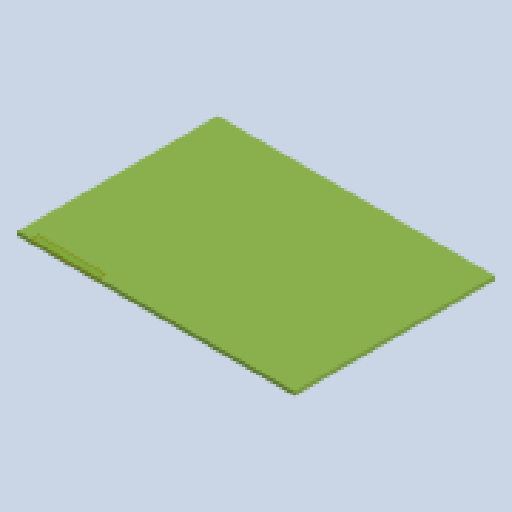
# Autodesk Inventor part: верхняя пластина
Saved by Autodesk Inventor 2024.2 (Build 282272000, 272)
## iProperties
Created: 2025-11-23
Part Number: верхняя пластина
Material: Типовые
Document SubType Name: Modeling
Designer: katya_notebook
Density: 1 g/cm^3
Appearance: Оливково-зеленый
Author: katya_notebook
Autodesk Inventor part; units mm, degrees
ref_plane "YZ Plane" through (0, 0, 0) normal (1, 0, 0) x (0, 1, 0)
ref_plane "XZ Plane" through (0, 0, 0) normal (0, 1, 0) x (-1, 0, 0)
ref_plane "XY Plane" through (0, 0, 0) normal (0, 0, 1) x (1, 0, 0)
ref_plane "РабПлоскость1" through (-492.61, -280.3956, -187.6025) normal (0, -1, 0) x (1, 0, 0)
sketch "Эскиз1" plane through (-492.61, -280.3956, -187.6025) normal (0, -1, 0) x (1, 0, 0)
  line L0 (-76.4763, 6.5) -> (193.5237, 6.5)
  line L1 (193.5237, 6.5) -> (193.5237, -188.5)
  line L2 (193.5237, -188.5) -> (-76.4763, -188.5)
  line L3 (-76.4763, -188.5) -> (-76.4763, 6.5)
  line L4 (-76.4763, -188.5) -> (-76.4763, 6.5) projected
  circle A0 centre (-12, 3.25) radius 1.75
  circle A1 centre (-48, 3.25) radius 1.75
  circle A2 centre (-30, 3.25) radius 1.75
  line L5 (-76.4763, -91) -> (193.5237, -91)
  circle A3 centre (-12, -185.25) radius 1.75
  circle A4 centre (-48, -185.25) radius 1.75
  circle A5 centre (-30, -185.25) radius 1.75
  point P0 (492.61, 187.6025)
  point P1 (-60, 3.25)
  dimension "d0" = 195
  dimension "d1" = 270
  dimension "d2" = 0
  dimension "d5" = 3.5
  dimension "d6" = 3.5
  dimension "d8" = 12
  dimension "d9" = 3.25
  dimension "d10" = 3.25
  dimension "d11" = 3.5
  dimension "d12" = 3.25
  dimension "d13" = 18
  dimension "d14" = 97.5
  constraints: 10 end point, 6 centre point, 3 symmetric about line, 2 midpoint, 2 parallel, 2 perpendicular, 1 horizontal, 3 other
  measures "d0" distance of L0.end L1.end
  measures "d1" distance of L1.end L2.end
  measures "d2" distance between parallel lines of L4 L3
  measures "d5" diameter of A1
  measures "d6" diameter of A0
  measures "d8" distance of A1.centre point (-60, 3.25)
  measures "d9" distance from line of L0 A0.centre
  measures "d10" distance from line of L0 A1.centre
  measures "d11" diameter of A2
  measures "d12" distance from line of L0 A2.centre
  measures "d13" distance of A1.centre A2.centre
  measures "d14" distance between parallel lines of L5 L0
extrude "Выдавливание1" add sketch "Эскиз1" along normal blind 4 contours L0 L1 L5 L3 | L5 L1 L2 L3 | A0 | A1 | A2 | A3 | A4 | A5
